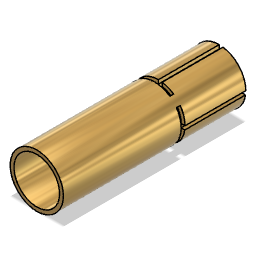
electrode puck v2 pulse plug v8 (Autodesk Fusion 360 design; units mm, degrees)
Autodesk Fusion 360 part; units mm, degrees
note: some values were not read from the file. Chosen so that the rebuilt part matches the saved one: that a step has no effect. Set by a fixed rule: which sketch regions a step uses.
sketch "Sketch1" plane through (0, 0, 0) normal (0, 1, 0) x (1, 0, 0)
  line L0 (0, 0) -> (0, -12)
  line L1 (0, -12) -> (1.75, -12)
  line L2 (1.75, -12) -> (1.75, 0)
  line L3 (1.75, 0) -> (0, 0)
  line L4 (1.5, 0) -> (1.5, -12)
  line L5 (0.25, 0) -> (0.25, -4)
  line L6 (0.25, -4) -> (0, -4)
  line L7 (-1, -4) -> (1, -4)
  line L8 (1, -4) -> (1, -4.25)
  line L9 (1, -4.25) -> (-1, -4.25)
  line L10 (-1, -4.25) -> (-1, -4)
  dimension "d2" = 0.25
  dimension "d4" = 0.25
  dimension "d5" = 4
  dimension "d8" = 0.25
  dimension "d9" = 2
  dimension "d15" = 12
  dimension "d18" = 1.5
  constraint coincident L0.start L3.end
  constraint vertical L0
  constraint perpendicular L0 L1
  constraint perpendicular L0 L3
  constraint coincident L3 L4.start
  constraint coincident L1 L4.end
  constraint perpendicular L1 L4
  constraint coincident L3 L5.start
  constraint perpendicular L3 L5
  constraint coincident L0 L6.end
  constraint perpendicular L0 L6
  constraint horizontal L7
  constraint vertical L8
  constraint horizontal L9
  constraint vertical L10
  constraint symmetric L0 L8 L10
  constraint collinear L6 L7
  measures "d2" distance of L2 L4
  measures "d4" distance of L0 L5
  measures "d5" distance of L5.start L5.end
  measures "d8" distance of L7.start L9.end
  measures "d9" distance of L8.end L9.end
  measures "d15" distance of L1 L3
  measures "d18" distance of L0 L4
revolve "Revolve1" add sketch "Sketch1" angle 360 about axis through (0, 0, 0) along (0, 0, 1) contours L1 L2 L3 L4
chamfer "Chamfer1" [no effect]
extrude "Extrude1" cut sketch "Sketch1" along normal blind 5 contours L0 L3 L5 L6 L7 | L0 L6 L7 L8 L9 | L0 L7 L9 L10
pattern_circular "C-Pattern1" count 4 over 360 about axis through (0, 0, 0) along (0, 0, 1) of "Extrude1"
